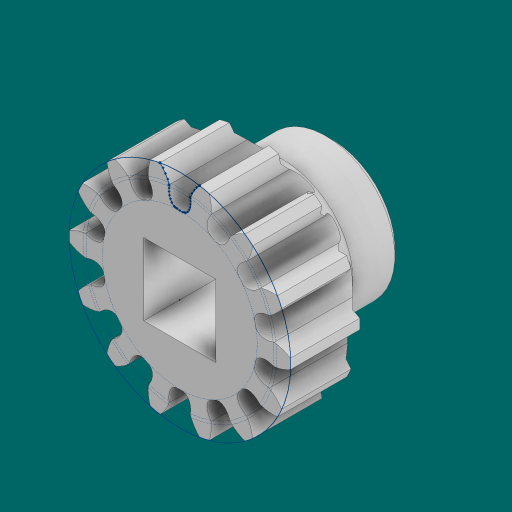
# Autodesk Inventor part: downcoming_spur
Saved by Autodesk Inventor 2023.1 (Build 271208000, 208)
## iProperties
Created: 2022-11-06
Part Number: downcoming_spur
Material: Generic
Document SubType Name: Modeling
Designer: zac-h
Density: 1 g/cm^3
Appearance: Default
Author: zac-h
## iProperties of the stored document downcoming_spur_3DPrint.ipt
Created: 2022-11-06
Part Number: downcoming_spur_3DPrint
Material: Generic
Document SubType Name: Modeling
Designer: zac-h
Density: 1 g/cm^3
Appearance: Default
Author: zac-h
Autodesk Inventor part; units mm, degrees
ref_plane "YZ Plane" through (0, 0, 0) normal (1, 0, 0) x (0, 1, 0)
ref_plane "XZ Plane" through (0, 0, 0) normal (0, 1, 0) x (-1, 0, 0)
ref_plane "XY Plane" through (0, 0, 0) normal (0, 0, 1) x (1, 0, 0)
sketch "Sketch1" plane through (0, 0, 0) normal (0, 0, 1) x (1, 0, 0)
  spline S0 degree 3 poles (-1.8138, 9.9968) (-1.7255, 9.8968) (-1.549, 9.6967) (-1.32, 9.3685) (-1.1164, 9.0224) (-1.0291, 8.7701) (-0.9855, 8.644) knots 0 0 0 0 0.250086 0.500175 0.75021 1 1 1 1
  spline S1 degree 3 poles (-0.9855, 8.644) (-0.9944, 8.5543) (-1.0123, 8.375) (-1.0082, 8.1041) (-0.9681, 7.8362) (-0.8859, 7.5772) (-0.7451, 7.3439) (-0.5715, 7.1921) (-0.4039, 7.124) (-0.2256, 7.0909) (0, 7.1108) (0.2256, 7.0909) (0.4039, 7.124) (0.5715, 7.1921) (0.7451, 7.3439) (0.8859, 7.5772) (0.9681, 7.8362) (1.0082, 8.1041) (1.0123, 8.375) (0.9944, 8.5543) (0.9855, 8.644) knots 0 0 0 0 0.062562 0.125127 0.18768 0.250213 0.312668 0.374984 0.406245 0.437411 0.5 0.562589 0.593755 0.625016 0.687332 0.749787 0.81232 0.874873 0.937438 1 1 1 1
  spline S2 degree 3 poles (0.9855, 8.644) (1.0291, 8.7701) (1.1164, 9.0224) (1.32, 9.3685) (1.549, 9.6967) (1.7255, 9.8968) (1.8138, 9.9968) knots 0 0 0 0 0.24979 0.499825 0.749914 1 1 1 1
  circle A0 centre (0, 0) radius 7.1028 construction
  circle A1 centre (0, 0) radius 8.6068 construction
  circle A2 centre (0, 0) radius 8.89 construction
  circle A3 centre (0, 0) radius 10.16
  point P0 (-1.555, 9.692)
  point P1 (-1.3242, 9.3654)
  point P2 (-1.1284, 9.0169)
  point P3 (-1.0071, 8.3747)
  point P4 (-1.0022, 8.1046)
  point P5 (-0.9611, 7.8376)
  point P6 (-0.8761, 7.5813)
  point P7 (-0.7337, 7.3522)
  point P8 (-0.5274, 7.1796)
  point P9 (-0.4025, 7.1283)
  point P10 (-0.2703, 7.1033)
  point P11 (0, 7.1028)
  point P12 (0.2703, 7.1033)
  point P13 (0.4025, 7.1283)
  point P14 (0.5274, 7.1796)
  point P15 (0.7337, 7.3522)
  point P16 (0.8761, 7.5813)
  point P17 (0.9611, 7.8376)
  point P18 (1.0022, 8.1046)
  point P19 (1.0071, 8.3747)
  point P20 (1.1284, 9.0169)
  point P21 (1.3242, 9.3654)
  point P22 (1.555, 9.692)
  constraints: 4 centre point, 2 point on circle, 61 other
extrude "Extrusion1" add sketch "Sketch1" against normal blind 6.35
extrude "Extrusion2" cut sketch "Sketch1" against normal through all contours A3 S2 S1 S0 picked at (0.2025, 9.1433)
pattern_circular "Circular Pattern1" count 14 over 360 about axis through (0, 0, 0) along (0, 0, -1) of "Extrusion2"
sketch "Sketch2" plane through (0, 0, 0) normal (0, 0, 1) x (1, 0, 0)
  point P0 (0, 0)
sketch "Sketch3" plane through (0, 0, 0) normal (0, 0, 1) x (1, 0, 0)
  line L0 (-3.302, 3.302) -> (3.302, 3.302)
  line L1 (3.302, 3.302) -> (3.302, -3.302)
  line L2 (3.302, -3.302) -> (-3.302, -3.302)
  line L3 (-3.302, -3.302) -> (-3.302, 3.302)
  line L4 (-3.302, 3.302) -> (3.302, -3.302) construction
  line L5 (3.302, 3.302) -> (-3.302, -3.302) construction
  point P0 (0, 0)
  dimension "d7" = 6.604
  dimension "d8" = 6.604
  constraints: 12 end point, 2 midpoint, 2 parallel, 1 horizontal, 1 perpendicular
  measures "d7" distance of L1.end L2.end
  measures "d8" distance of L0.end L1.end
extrude "Extrusion3" cut sketch "Sketch3" against normal through all
sketch "Sketch5" plane through (0, 0, -6.35) normal (0, 0, -1) x (-1, 0, 0)
  circle A0 centre (0, 0) radius 6.35
  line L0 (-3.302, 3.302) -> (3.302, 3.302) projected
  line L1 (-3.302, -3.302) -> (3.302, -3.302)
  line L2 (3.302, -3.302) -> (3.302, 3.302)
  line L3 (3.302, 3.302) -> (-3.302, 3.302)
  line L4 (-3.302, 3.302) -> (-3.302, -3.302)
  line L5 (-3.302, -3.302) -> (3.302, 3.302) construction
  line L6 (3.302, -3.302) -> (-3.302, 3.302) construction
  dimension "d15" = 12.7
  constraints: 12 end point, 2 midpoint, 2 parallel, 1 centre point, 1 coincident, 1 horizontal, 1 perpendicular
  measures "d15" diameter of A0
extrude "Extrusion5" add sketch "Sketch5" along normal blind 7.62
chamfer "Chamfer1" distance 3.175 angle 45 1 edges at (6.35, 0, -6.35)
chamfer "Chamfer2" distance 0.6 angle 45 1 edges at (6.35, 0, -13.97)
sketch "Sketch6" plane through (0, 0, -13.97) normal (0, 0, -1) x (-1, 0, 0)
  line L0 (-1.651, -1.651) -> (1.651, -1.651)
  line L1 (1.651, -1.651) -> (1.651, 1.651)
  line L2 (1.651, 1.651) -> (-1.651, 1.651)
  line L3 (-1.651, 1.651) -> (-1.651, -1.651)
  line L4 (-1.651, -1.651) -> (1.651, 1.651) construction
  line L5 (1.651, -1.651) -> (-1.651, 1.651) construction
  line L6 (-3.302, -3.302) -> (3.302, -3.302)
  line L7 (3.302, -3.302) -> (3.302, 3.302)
  line L8 (3.302, 3.302) -> (-3.302, 3.302)
  line L9 (-3.302, 3.302) -> (-3.302, -3.302)
  line L10 (-3.302, -3.302) -> (3.302, 3.302) construction
  line L11 (3.302, -3.302) -> (-3.302, 3.302) construction
  point P0 (0, 0)
  dimension "d24" = 3.302
  dimension "d25" = 3.302
  constraints: 24 end point, 4 midpoint, 4 parallel, 2 horizontal, 2 perpendicular
  measures "d24" distance of L2.end L1.end
  measures "d25" distance of L1.end L0.end
extrude "Extrusion6" add sketch "Sketch6" against normal blind 2.54
equation "\"d0\" = FaceWidth"
equation "\"Module\" = 1.27"
equation "\"PressureAngle\" = 14.5deg"
equation "\"UnitProfileClearance\" = 0.25"
equation "\"UnitRoundRadius\" = 0.3335"
equation "\"HeadDiameter\" = 20.32"
equation "\"RootDiameter\" = 14.20561"
equation "\"BaseDiameter\" = 17.21367"
equation "\"PitchDiameter\" = 17.78"
equation "\"FaceWidth\" = 6.35"
equation "\"HelixAngle\" = 0"
equation "\"UnitCorrection\" = 0"
equation "\"UnitAddendumModification\" = 0"
equation "\"CircularPitch\" = 3.98982"
equation "\"UnitBacklashShift\" = -0.157241"
equation "\"TotalToolShift\" = -0.1997"
equation "\"IsInternal\" = 0"
body "Solid1"
